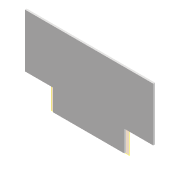
# Autodesk Inventor part: tussenschotje
Saved by Autodesk Inventor 2020.3 (Build 243373000, 373)
## iProperties
Created: 2020-11-26
Part Number: tussenschotje
Material: Wood (Birch)
Document SubType Name: Sheet Metal
Designer: Svend
Density: 0.55 g/cm^3
Sheet Metal Rule: Default_mm
Appearance: Birch - Natural Polished
Author: Svend
Autodesk Inventor part; units mm, degrees
ref_plane "YZ Plane" through (0, 0, 0) normal (1, 0, 0) x (0, 1, 0)
ref_plane "XZ Plane" through (0, 0, 0) normal (0, 1, 0) x (-1, 0, 0)
ref_plane "XY Plane" through (0, 0, 0) normal (0, 0, 1) x (1, 0, 0)
ref_plane "Work Plane1" through (0, 0, 0) normal (0, 0, 1) x (1, 0, 0)
sketch "Sketch1" plane through (0, 0, 0) normal (0, 0, 1) x (1, 0, 0)
  line L0 (0, 0) -> (20, 0)
  line L1 (0, 0) -> (0, -6)
  line L2 (20, -6) -> (0, -6)
  line L3 (20, 0) -> (20, -6)
  line L4 (34.15, 0) -> (34.15, 6.2)
  line L5 (34.15, 0) -> (28.15, 0)
  line L6 (28.15, 6.2) -> (28.15, 0)
  line L7 (34.15, 6.2) -> (28.15, 6.2)
  line L8 (28.15, 15) -> (28.15, 0)
  line L9 (-7.85, 48.6) -> (-7.85, 2.8)
  line L10 (-7.85, 0) -> (28.15, 0)
  line L11 (28.15, 0) -> (28.15, 15)
  line L12 (28.15, 15) -> (-7.85, 15)
  line L13 (-7.85, 15) -> (-7.85, 0)
  line L14 (28.15, 15) -> (-7.85, 31.05)
  line L15 (-7.85, 31.05) -> (-7.85, 15)
  line L16 (-6.35, 0) -> (-6.35, 30.3813)
  point P0 (-8.95, 31.05)
  dimension "d1" = 1.5
  measures "d1" distance between parallel lines of L9 L16
extrude "Plate2" add sketch "Sketch1" along normal blind 6 contours L10 L16 L12 L8 L6 L0 | L0 L3 L2 L1 | L16 L14 L12
equation "\"d2\" = Thickness"
equation "\"BendRadius\" = Thickness"
equation "\"BendReliefWidth\" = Thickness"
equation "\"BendReliefDepth\" = 0.5 * Thickness"
equation "\"CornerReliefSize\" = 4 * Thickness"
equation "\"MinimumRemnant\" = 2 * Thickness"
equation "\"TransitionRadius\" = BendRadius"
equation "\"JacobiRadiusSize\" = BendRadius"
equation "\"GapSize\" = Thickness"
equation "\"Thickness\" = 6"
body "Solid2"
